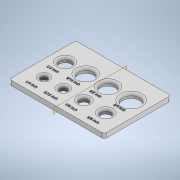
# Autodesk Inventor part: inchHexSocketSetOf8
Saved by Autodesk Inventor 2020.3 (Build 243373000, 373)
## iProperties
Created: 2020-03-13
Part Number: inchHexSocketSetOf8
Material: Generic
Document SubType Name: Modeling
Designer: robst
Density: 1 g/cm^3
Appearance: Default
Author: robst
Autodesk Inventor part; units mm, degrees
(part 1 of 2)
ref_plane "XZ Plane" through (0, 0, 0) normal (0, 1, 0) x (-1, 0, 0)
ref_plane "XY Plane" through (0, 0, 0) normal (0, 0, 1) x (1, 0, 0)
sketch "Sketch1" plane through (0, 0, 0) normal (0, 1, 0) x (-1, 0, 0)
  line L0 (63.5, 44.45) -> (-63.5, 44.45)
  line L1 (-63.5, 44.45) -> (-63.5, -44.45)
  line L2 (-63.5, -44.45) -> (63.5, -44.45)
  line L3 (63.5, -44.45) -> (63.5, 44.45)
  line L4 (63.5, 44.45) -> (-63.5, -44.45) construction
  line L5 (-63.5, 44.45) -> (63.5, -44.45) construction
  point P0 (0, 0)
  dimension "d3" = 88.9
  dimension "d13" = 127
  constraints: 12 end point, 2 midpoint, 2 parallel, 1 horizontal, 1 perpendicular
  measures "d3" distance of L2.end L0.start
  measures "d13" distance of L1.end L2.end
extrude "Extrusion1" add sketch "Sketch1" against normal blind 6.35
sketch "Sketch4" plane through (0, 0, 0) normal (0, 1, 0) x (1, 0, 0)
  line L0 (-63.5, -44.45) -> (-63.5, 44.45) construction
  line L1 (-63.5, -19.05) -> (63.5, -19.05) construction
  line L2 (63.5, 44.45) -> (63.5, -44.45) construction
  line L3 (-63.5, -44.45) -> (63.5, -44.45) projected
  circle A0 centre (-42.4637, -19.05) radius 4.318
  circle A1 centre (-16.6014, -19.05) radius 4.826
  circle A2 centre (10.7848, -19.05) radius 5.842
  circle A3 centre (40.0761, -19.05) radius 6.731
  line L4 (-63.5, 12.7) -> (63.5, 12.7) construction
  circle A4 centre (-45.9232, 12.7) radius 7.874
  circle A5 centre (-18.3134, 12.7) radius 10.033
  circle A6 centre (11.3284, 12.7) radius 9.906
  circle A7 centre (42.3672, 12.7) radius 11.43
  point P0 (0, 0)
  dimension "d16" = 25.4
  dimension "hex1_4inchHole" = 8.636
  dimension "gap0" = 16.7183
  dimension "hex5_16inchHole" = 9.652
  dimension "gap1" = 25.8623
  dimension "hex3_8inchHole" = 11.684
  dimension "gap2" = 27.3863
  dimension "gap3" = 29.2913
  dimension "hex7_16inchHole" = 13.462
  dimension "frontToBackRowGap" = 31.75
  dimension "gap5" = 9.7028
  dimension "hex1_2inchHole" = 15.748
  dimension "hex9_16inchHole" = 20.066
  dimension "gap6" = 27.6098
  dimension "hex5_8inchHole" = 19.812
  dimension "gap7" = 29.6418
  dimension "hex3_4inchHole" = 22.86
  dimension "gap8" = 31.0388
  dimension "d37" = 9.7028
  dimension "d57" = 16.6929
  constraints: 12 point on line, 8 centre point, 4 end point, 1 horizontal, 1 perpendicular
  measures "d16" distance between parallel lines of L1 L3
  measures "hex1_4inchHole" diameter of A0
  measures "gap0" distance edge to line of A0 L0
  measures "hex5_16inchHole" diameter of A1
  measures "gap1" distance of A1.centre A0.centre
  measures "hex3_8inchHole" diameter of A2
  measures "gap2" distance of A2.centre A1.centre
  measures "gap3" distance of A3.centre A2.centre
  measures "hex7_16inchHole" diameter of A3
  measures "frontToBackRowGap" distance between parallel lines of L4 L1
  measures "gap5" distance edge to line of A4 L0
  measures "hex1_2inchHole" diameter of A4
  measures "hex9_16inchHole" diameter of A5
  measures "gap6" distance of A5.centre A4.centre
  measures "hex5_8inchHole" diameter of A6
  measures "gap7" distance of A6.centre A5.centre
  measures "hex3_4inchHole" diameter of A7
  measures "gap8" distance of A7.centre A6.centre
  measures "d37" distance edge to line of A7 L2
  measures "d57" distance edge to line of A3 L2
extrude "Extrusion3" cut sketch "Sketch4" against normal through all
sketch "Sketch7" plane through (0, 0, 0) normal (0, 1, 0) x (1, 0, 0)
  circle A0 centre (-42.4637, -19.05) radius 4.318 construction
  line L0 (63.5, -44.45) -> (-63.5, -44.45) construction
  line L1 (-46.7817, -35.6779) -> (-38.1457, -35.6779) construction
  line L2 (-21.4274, -35.6779) -> (-11.7754, -35.6779) construction
  line L3 (4.9428, -35.6779) -> (16.6268, -35.6779) construction
  line L4 (33.3451, -35.6779) -> (46.8071, -35.6779) construction
  line L5 (-53.7972, -3.81) -> (-38.0492, -3.81) construction
  line L6 (-28.3464, -3.9984) -> (-8.2804, -3.9984) construction
  line L7 (1.4224, -3.8276) -> (21.2344, -3.8276) construction
  line L8 (30.9372, -3.6244) -> (55.5752, -3.6244) construction
  line L9 (-21.4274, -35.6779) -> (-21.4274, -19.05) construction
  circle A1 centre (-16.6014, -19.05) radius 4.826 construction
  line L10 (-11.7754, -35.6779) -> (-11.7754, -19.05) construction
  line L11 (-46.7817, -19.05) -> (-46.7817, -35.6779) construction
  line L12 (-38.1457, -35.6779) -> (-38.1457, -19.05) construction
  line L13 (4.9428, -35.6779) -> (4.9428, -19.05) construction
  circle A2 centre (10.7848, -19.05) radius 5.842 construction
  line L14 (16.6268, -35.6779) -> (16.6268, -19.05) construction
  line L15 (46.8071, -35.6779) -> (46.8071, -19.05) construction
  circle A3 centre (40.0761, -19.05) radius 6.731 construction
  line L16 (33.3451, -35.6779) -> (33.3451, -19.05) construction
  circle A4 centre (-45.9232, 12.7) radius 7.874 construction
  line L17 (-53.7972, 12.7) -> (-53.7972, -3.81) construction
  line L18 (-38.0492, 12.7) -> (-38.0492, -3.81) construction
  circle A5 centre (-18.3134, 12.7) radius 10.033 construction
  line L19 (-28.3464, 12.7) -> (-28.3464, -3.9984) construction
  line L20 (-8.2804, 12.7) -> (-8.2804, -3.9984) construction
  circle A6 centre (11.3284, 12.7) radius 9.906 construction
  line L21 (1.4224, 12.7) -> (1.4224, -3.8276) construction
  line L22 (21.2344, 12.7) -> (21.2344, -3.8276) construction
  circle A7 centre (42.3672, 12.7) radius 11.43 construction
  line L23 (30.9372, 12.7) -> (30.9372, -3.6244) construction
  line L24 (55.5752, 12.702) -> (55.5752, -3.6244) construction
  line L25 (-51.5005, -5.334) -> (-52.9874, -5.334)
  line L26 (-52.9874, -5.334) -> (-52.9874, -5.0228)
  line L27 (-52.9874, -5.0228) -> (-52.4342, -5.0228)
  line L28 (-52.4342, -5.0228) -> (-52.4342, -2.9801)
  line L29 (-52.4342, -2.9801) -> (-52.9874, -2.9801)
  line L30 (-52.9874, -2.9801) -> (-52.9874, -2.701)
  spline S0 degree 2 poles (-52.9874, -2.701) (-52.6738, -2.701) (-52.3774, -2.5231) (-52.3576, -2.2761) knots 0 0 0 1 2 2 2
  line L31 (-52.3576, -2.2761) -> (-52.0414, -2.2761)
  line L32 (-52.0414, -2.2761) -> (-52.0414, -5.0228)
  line L33 (-52.0414, -5.0228) -> (-51.5005, -5.0228)
  line L34 (-51.5005, -5.0228) -> (-51.5005, -5.334)
  line L35 (-49.6727, -2.1501) -> (-50.8657, -5.996)
  line L36 (-50.8657, -5.996) -> (-51.2115, -5.996)
  line L37 (-51.2115, -5.996) -> (-50.0234, -2.1501)
  line L38 (-50.0234, -2.1501) -> (-49.6727, -2.1501)
  line L39 (-47.4571, -5.334) -> (-49.3368, -5.334)
  line L40 (-49.3368, -5.334) -> (-49.3368, -4.9017)
  spline S1 degree 2 poles (-49.3368, -4.9017) (-49.1342, -4.7116) (-48.7736, -4.3583) (-48.6007, -4.1682) knots 0 0 0 1 2 2 2
  spline S2 degree 2 poles (-48.6007, -4.1682) (-48.2524, -3.7853) (-47.998, -3.3259) (-47.998, -3.0813) knots 0 0 0 1 2 2 2
  spline S3 degree 2 poles (-47.998, -3.0813) (-47.998, -2.9529) (-48.0771, -2.7602) (-48.1487, -2.6985) knots 0 0 0 1 2 2 2
  spline S4 degree 2 poles (-48.1487, -2.6985) (-48.2203, -2.6367) (-48.408, -2.575) (-48.5217, -2.575) knots 0 0 0 1 2 2 2
  spline S5 degree 2 poles (-48.5217, -2.575) (-48.6303, -2.575) (-48.8526, -2.6293) (-48.9539, -2.6713) knots 0 0 0 1 2 2 2
  spline S6 degree 2 poles (-48.9539, -2.6713) (-49.0404, -2.7059) (-49.2009, -2.8047) (-49.2503, -2.8393) knots 0 0 0 1 2 2 2
  line L41 (-49.2503, -2.8393) -> (-49.2725, -2.8393)
  line L42 (-49.2725, -2.8393) -> (-49.2725, -2.4046)
  spline S7 degree 2 poles (-49.2725, -2.4046) (-49.1466, -2.3428) (-48.6946, -2.2218) (-48.492, -2.2218) knots 0 0 0 1 2 2 2
  spline S8 degree 2 poles (-48.492, -2.2218) (-48.0647, -2.2218) (-47.5831, -2.6738) (-47.5831, -3.0591) knots 0 0 0 1 2 2 2
  spline S9 degree 2 poles (-47.5831, -3.0591) (-47.5831, -3.2394) (-47.667, -3.5408) (-47.7411, -3.6692) knots 0 0 0 1 2 2 2
  spline S10 degree 2 poles (-47.7411, -3.6692) (-47.8152, -3.8026) (-48.0301, -4.0644) (-48.1487, -4.1904) knots 0 0 0 1 2 2 2
  spline S11 degree 2 poles (-48.1487, -4.1904) (-48.3413, -4.4003) (-48.8131, -4.8499) (-48.9539, -4.9808) knots 0 0 0 1 2 2 2
  line L43 (-48.9539, -4.9808) -> (-47.4571, -4.9808)
  line L44 (-47.4571, -4.9808) -> (-47.4571, -5.334)
  line L45 (-45.2909, -5.334) -> (-45.6762, -5.334)
  line L46 (-45.6762, -5.334) -> (-45.6762, -3.0468)
  line L47 (-45.6762, -3.0468) -> (-45.2909, -3.0468)
  line L48 (-45.2909, -3.0468) -> (-45.2909, -5.334)
  line L49 (-45.2637, -2.6664) -> (-45.7009, -2.6664)
  line L50 (-45.7009, -2.6664) -> (-45.7009, -2.2662)
  line L51 (-45.7009, -2.2662) -> (-45.2637, -2.2662)
  line L52 (-45.2637, -2.2662) -> (-45.2637, -2.6664)
  line L53 (-42.9295, -5.334) -> (-43.3149, -5.334)
  line L54 (-43.3149, -5.334) -> (-43.3149, -4.0298)
  spline S12 degree 2 poles (-43.3149, -4.0298) (-43.3149, -3.8718) (-43.3445, -3.6) (-43.389, -3.5185) knots 0 0 0 1 2 2 2
  spline S13 degree 2 poles (-43.389, -3.5185) (-43.4359, -3.4321) (-43.6039, -3.3481) (-43.7471, -3.3481) knots 0 0 0 1 2 2 2
  spline S14 degree 2 poles (-43.7471, -3.3481) (-43.8904, -3.3481) (-44.1942, -3.5012) (-44.3399, -3.6247) knots 0 0 0 1 2 2 2
  line L55 (-44.3399, -3.6247) -> (-44.3399, -5.334)
  line L56 (-44.3399, -5.334) -> (-44.7252, -5.334)
  line L57 (-44.7252, -5.334) -> (-44.7252, -3.0468)
  line L58 (-44.7252, -3.0468) -> (-44.3399, -3.0468)
  line L59 (-44.3399, -3.0468) -> (-44.3399, -3.3012)
  spline S15 degree 2 poles (-44.3399, -3.3012) (-44.167, -3.1456) (-43.8336, -2.9825) (-43.6458, -2.9825) knots 0 0 0 1 2 2 2
  spline S16 degree 2 poles (-43.6458, -2.9825) (-43.3099, -2.9825) (-42.9295, -3.4271) (-42.9295, -3.8495) knots 0 0 0 1 2 2 2
  line L60 (-42.9295, -3.8495) -> (-42.9295, -5.334)
  spline S17 degree 2 poles (-41.4796, -5.3859) (-41.7168, -5.3859) (-42.1095, -5.2401) (-42.2503, -5.0919) knots 0 0 0 1 2 2 2
  spline S18 degree 2 poles (-42.2503, -5.0919) (-42.3911, -4.9462) (-42.5467, -4.4967) (-42.5467, -4.1953) knots 0 0 0 1 2 2 2
  spline S19 degree 2 poles (-42.5467, -4.1953) (-42.5467, -3.894) (-42.3861, -3.4543) (-42.2503, -3.3061) knots 0 0 0 1 2 2 2
  spline S20 degree 2 poles (-42.2503, -3.3061) (-42.1144, -3.1554) (-41.7118, -2.9949) (-41.4796, -2.9949) knots 0 0 0 1 2 2 2
  spline S21 degree 2 poles (-41.4796, -2.9949) (-41.2919, -2.9949) (-40.9412, -3.1011) (-40.8053, -3.1703) knots 0 0 0 1 2 2 2
  line L61 (-40.8053, -3.1703) -> (-40.8053, -3.6025)
  line L62 (-40.8053, -3.6025) -> (-40.8276, -3.6025)
  spline S22 degree 2 poles (-40.8276, -3.6025) (-40.8695, -3.5679) (-40.998, -3.479) (-41.0894, -3.4321) knots 0 0 0 1 2 2 2
  spline S23 degree 2 poles (-41.0894, -3.4321) (-41.1709, -3.3926) (-41.3883, -3.3308) (-41.4871, -3.3308) knots 0 0 0 1 2 2 2
  spline S24 degree 2 poles (-41.4871, -3.3308) (-41.7859, -3.3308) (-42.149, -3.7828) (-42.149, -4.1953) knots 0 0 0 1 2 2 2
  spline S25 degree 2 poles (-42.149, -4.1953) (-42.149, -4.5979) (-41.7983, -5.0499) (-41.4871, -5.0499) knots 0 0 0 1 2 2 2
  spline S26 degree 2 poles (-41.4871, -5.0499) (-41.2993, -5.0499) (-40.9585, -4.8943) (-40.8276, -4.7733) knots 0 0 0 1 2 2 2
  line L63 (-40.8276, -4.7733) -> (-40.8053, -4.7733)
  line L64 (-40.8053, -4.7733) -> (-40.8053, -5.2056)
  spline S27 degree 2 poles (-40.8053, -5.2056) (-40.8621, -5.2327) (-41.035, -5.3093) (-41.1042, -5.3266) knots 0 0 0 1 2 2 2
  spline S28 degree 2 poles (-41.1042, -5.3266) (-41.203, -5.3562) (-41.3586, -5.3859) (-41.4796, -5.3859) knots 0 0 0 1 2 2 2
  line L65 (-38.6589, -5.334) -> (-39.0442, -5.334)
  line L66 (-39.0442, -5.334) -> (-39.0442, -4.0298)
  spline S29 degree 2 poles (-39.0442, -4.0298) (-39.0442, -3.8718) (-39.0738, -3.6) (-39.1183, -3.5185) knots 0 0 0 1 2 2 2
  spline S30 degree 2 poles (-39.1183, -3.5185) (-39.1652, -3.4321) (-39.3332, -3.3481) (-39.4765, -3.3481) knots 0 0 0 1 2 2 2
  spline S31 degree 2 poles (-39.4765, -3.3481) (-39.6197, -3.3481) (-39.9235, -3.5012) (-40.0693, -3.6247) knots 0 0 0 1 2 2 2
  line L67 (-40.0693, -3.6247) -> (-40.0693, -5.334)
  line L68 (-40.0693, -5.334) -> (-40.4546, -5.334)
  line L69 (-40.4546, -5.334) -> (-40.4546, -2.1501)
  line L70 (-40.4546, -2.1501) -> (-40.0693, -2.1501)
  line L71 (-40.0693, -2.1501) -> (-40.0693, -3.3012)
  spline S32 degree 2 poles (-40.0693, -3.3012) (-39.8964, -3.1456) (-39.5629, -2.9825) (-39.3752, -2.9825) knots 0 0 0 1 2 2 2
  spline S33 degree 2 poles (-39.3752, -2.9825) (-39.0393, -2.9825) (-38.6589, -3.4271) (-38.6589, -3.8495) knots 0 0 0 1 2 2 2
  line L72 (-38.6589, -3.8495) -> (-38.6589, -5.334)
  spline S34 degree 2 poles (-26.8448, -3.4649) (-26.8448, -3.2303) (-26.6917, -2.84) (-26.5583, -2.6992) knots 0 0 0 1 2 2 2
  spline S35 degree 2 poles (-26.5583, -2.6992) (-26.4323, -2.5634) (-26.0643, -2.4127) (-25.8766, -2.4127) knots 0 0 0 1 2 2 2
  spline S36 degree 2 poles (-25.8766, -2.4127) (-25.6666, -2.4127) (-25.3258, -2.5535) (-25.1998, -2.6869) knots 0 0 0 1 2 2 2
  spline S37 degree 2 poles (-25.1998, -2.6869) (-25.0417, -2.8548) (-24.8688, -3.3982) (-24.8688, -3.8157) knots 0 0 0 1 2 2 2
  spline S38 degree 2 poles (-24.8688, -3.8157) (-24.8688, -4.1936) (-25.0393, -4.8704) (-25.2047, -5.0951) knots 0 0 0 1 2 2 2
  spline S39 degree 2 poles (-25.2047, -5.0951) (-25.3801, -5.3323) (-25.8741, -5.5817) (-26.2347, -5.5817) knots 0 0 0 1 2 2 2
  spline S40 degree 2 poles (-26.2347, -5.5817) (-26.3163, -5.5817) (-26.5015, -5.5644) (-26.5805, -5.5397) knots 0 0 0 1 2 2 2
  line L73 (-26.5805, -5.5397) -> (-26.5805, -5.147)
  line L74 (-26.5805, -5.147) -> (-26.5608, -5.147)
  spline S41 degree 2 poles (-26.5608, -5.147) (-26.5089, -5.1766) (-26.2916, -5.2285) (-26.1804, -5.2285) knots 0 0 0 1 2 2 2
  spline S42 degree 2 poles (-26.1804, -5.2285) (-25.7803, -5.2285) (-25.3233, -4.6999) (-25.2912, -4.2109) knots 0 0 0 1 2 2 2
  spline S43 degree 2 poles (-25.2912, -4.2109) (-25.4542, -4.322) (-25.7506, -4.4233) (-25.926, -4.4233) knots 0 0 0 1 2 2 2
  spline S44 degree 2 poles (-25.926, -4.4233) (-26.094, -4.4233) (-26.3731, -4.3492) (-26.5139, -4.243) knots 0 0 0 1 2 2 2
  spline S45 degree 2 poles (-26.5139, -4.243) (-26.6769, -4.117) (-26.8448, -3.7342) (-26.8448, -3.4649) knots 0 0 0 1 2 2 2
  spline S46 degree 2 poles (-25.2813, -3.7243) (-25.2813, -3.4155) (-25.3949, -3.0253) (-25.4962, -2.9191) knots 0 0 0 1 2 2 2
  spline S47 degree 2 poles (-25.4962, -2.9191) (-25.5851, -2.8202) (-25.7704, -2.7461) (-25.8791, -2.7461) knots 0 0 0 1 2 2 2
  spline S48 degree 2 poles (-25.8791, -2.7461) (-26.131, -2.7461) (-26.4299, -3.1068) (-26.4299, -3.4476) knots 0 0 0 1 2 2 2
  spline S49 degree 2 poles (-26.4299, -3.4476) (-26.4299, -3.6403) (-26.3311, -3.8898) (-26.2224, -3.9787) knots 0 0 0 1 2 2 2
  spline S50 degree 2 poles (-26.2224, -3.9787) (-26.1434, -4.0429) (-25.9482, -4.0849) (-25.8346, -4.0849) knots 0 0 0 1 2 2 2
  spline S51 degree 2 poles (-25.8346, -4.0849) (-25.7037, -4.0849) (-25.4023, -3.9935) (-25.2887, -3.9169) knots 0 0 0 1 2 2 2
  spline S52 degree 2 poles (-25.2887, -3.9169) (-25.2863, -3.8873) (-25.2813, -3.786) (-25.2813, -3.7243) knots 0 0 0 1 2 2 2
  line L75 (-23.2065, -2.3386) -> (-24.3995, -6.1844)
  line L76 (-24.3995, -6.1844) -> (-24.7453, -6.1844)
  line L77 (-24.7453, -6.1844) -> (-23.5572, -2.3386)
  line L78 (-23.5572, -2.3386) -> (-23.2065, -2.3386)
  line L79 (-21.144, -5.5224) -> (-22.631, -5.5224)
  line L80 (-22.631, -5.5224) -> (-22.631, -5.2112)
  line L81 (-22.631, -5.2112) -> (-22.0777, -5.2112)
  line L82 (-22.0777, -5.2112) -> (-22.0777, -3.1685)
  line L83 (-22.0777, -3.1685) -> (-22.631, -3.1685)
  line L84 (-22.631, -3.1685) -> (-22.631, -2.8894)
  spline S53 degree 2 poles (-22.631, -2.8894) (-22.3173, -2.8894) (-22.0209, -2.7116) (-22.0011, -2.4646) knots 0 0 0 1 2 2 2
  line L85 (-22.0011, -2.4646) -> (-21.685, -2.4646)
  line L86 (-21.685, -2.4646) -> (-21.685, -5.2112)
  line L87 (-21.685, -5.2112) -> (-21.144, -5.2112)
  line L88 (-21.144, -5.2112) -> (-21.144, -5.5224)
  spline S54 degree 2 poles (-18.6567, -4.5344) (-18.6567, -4.7691) (-18.8123, -5.1668) (-18.9433, -5.3001) knots 0 0 0 1 2 2 2
  spline S55 degree 2 poles (-18.9433, -5.3001) (-19.0791, -5.4409) (-19.42, -5.5867) (-19.625, -5.5867) knots 0 0 0 1 2 2 2
  spline S56 degree 2 poles (-19.625, -5.5867) (-19.83, -5.5867) (-20.1684, -5.4483) (-20.2968, -5.31) knots 0 0 0 1 2 2 2
  spline S57 degree 2 poles (-20.2968, -5.31) (-20.4549, -5.1445) (-20.6327, -4.5888) (-20.6327, -4.1837) knots 0 0 0 1 2 2 2
  spline S58 degree 2 poles (-20.6327, -4.1837) (-20.6327, -3.786) (-20.4697, -3.1463) (-20.2993, -2.9092) knots 0 0 0 1 2 2 2
  spline S59 degree 2 poles (-20.2993, -2.9092) (-20.1338, -2.677) (-19.6102, -2.4176) (-19.2668, -2.4176) knots 0 0 0 1 2 2 2
  spline S60 degree 2 poles (-19.2668, -2.4176) (-19.1656, -2.4176) (-18.9877, -2.4374) (-18.921, -2.4596) knots 0 0 0 1 2 2 2
  line L89 (-18.921, -2.4596) -> (-18.921, -2.8524)
  line L90 (-18.921, -2.8524) -> (-18.9383, -2.8524)
  spline S61 degree 2 poles (-18.9383, -2.8524) (-18.9951, -2.8227) (-19.2026, -2.7708) (-19.3212, -2.7708) knots 0 0 0 1 2 2 2
  spline S62 degree 2 poles (-19.3212, -2.7708) (-19.7015, -2.7708) (-20.1684, -3.2846) (-20.2128, -3.7885) knots 0 0 0 1 2 2 2
  spline S63 degree 2 poles (-20.2128, -3.7885) (-20.0671, -3.6872) (-19.7608, -3.5761) (-19.578, -3.5761) knots 0 0 0 1 2 2 2
  spline S64 degree 2 poles (-19.578, -3.5761) (-19.4002, -3.5761) (-19.1334, -3.6477) (-18.9877, -3.7564) knots 0 0 0 1 2 2 2
  spline S65 degree 2 poles (-18.9877, -3.7564) (-18.8198, -3.8824) (-18.6567, -4.2726) (-18.6567, -4.5344) knots 0 0 0 1 2 2 2
  spline S66 degree 2 poles (-19.0717, -4.5517) (-19.0717, -4.364) (-19.1705, -4.1096) (-19.2792, -4.0207) knots 0 0 0 1 2 2 2
  spline S67 degree 2 poles (-19.2792, -4.0207) (-19.3607, -3.9565) (-19.5632, -3.9145) (-19.6694, -3.9145) knots 0 0 0 1 2 2 2
  spline S68 degree 2 poles (-19.6694, -3.9145) (-19.8127, -3.9145) (-20.0819, -4.0009) (-20.2128, -4.0824) knots 0 0 0 1 2 2 2
  spline S69 degree 2 poles (-20.2128, -4.0824) (-20.2153, -4.1269) (-20.2203, -4.2109) (-20.2203, -4.2751) knots 0 0 0 1 2 2 2
  spline S70 degree 2 poles (-20.2203, -4.2751) (-20.2203, -4.5913) (-20.0968, -4.979) (-20.0029, -5.0803) knots 0 0 0 1 2 2 2
  spline S71 degree 2 poles (-20.0029, -5.0803) (-19.9164, -5.1766) (-19.7287, -5.2532) (-19.6225, -5.2532) knots 0 0 0 1 2 2 2
  spline S72 degree 2 poles (-19.6225, -5.2532) (-19.3755, -5.2532) (-19.0717, -4.9025) (-19.0717, -4.5517) knots 0 0 0 1 2 2 2
  line L91 (-16.5375, -5.5224) -> (-16.9228, -5.5224)
  line L92 (-16.9228, -5.5224) -> (-16.9228, -3.2352)
  line L93 (-16.9228, -3.2352) -> (-16.5375, -3.2352)
  line L94 (-16.5375, -3.2352) -> (-16.5375, -5.5224)
  line L95 (-16.5103, -2.8548) -> (-16.9475, -2.8548)
  line L96 (-16.9475, -2.8548) -> (-16.9475, -2.4547)
  line L97 (-16.9475, -2.4547) -> (-16.5103, -2.4547)
  line L98 (-16.5103, -2.4547) -> (-16.5103, -2.8548)
  line L99 (-14.1761, -5.5224) -> (-14.5614, -5.5224)
  line L100 (-14.5614, -5.5224) -> (-14.5614, -4.2183)
  spline S73 degree 2 poles (-14.5614, -4.2183) (-14.5614, -4.0602) (-14.5911, -3.7885) (-14.6355, -3.707) knots 0 0 0 1 2 2 2
  spline S74 degree 2 poles (-14.6355, -3.707) (-14.6825, -3.6205) (-14.8504, -3.5366) (-14.9937, -3.5366) knots 0 0 0 1 2 2 2
  spline S75 degree 2 poles (-14.9937, -3.5366) (-15.137, -3.5366) (-15.4408, -3.6897) (-15.5865, -3.8132) knots 0 0 0 1 2 2 2
  line L101 (-15.5865, -3.8132) -> (-15.5865, -5.5224)
  line L102 (-15.5865, -5.5224) -> (-15.9718, -5.5224)
  line L103 (-15.9718, -5.5224) -> (-15.9718, -3.2352)
  line L104 (-15.9718, -3.2352) -> (-15.5865, -3.2352)
  line L105 (-15.5865, -3.2352) -> (-15.5865, -3.4896)
  spline S76 degree 2 poles (-15.5865, -3.4896) (-15.4136, -3.334) (-15.0801, -3.171) (-14.8924, -3.171) knots 0 0 0 1 2 2 2
  spline S77 degree 2 poles (-14.8924, -3.171) (-14.5565, -3.171) (-14.1761, -3.6156) (-14.1761, -4.038) knots 0 0 0 1 2 2 2
  line L106 (-14.1761, -4.038) -> (-14.1761, -5.5224)
  spline S78 degree 2 poles (-12.7262, -5.5743) (-12.9633, -5.5743) (-13.3561, -5.4286) (-13.4969, -5.2804) knots 0 0 0 1 2 2 2
  spline S79 degree 2 poles (-13.4969, -5.2804) (-13.6377, -5.1347) (-13.7933, -4.6851) (-13.7933, -4.3838) knots 0 0 0 1 2 2 2
  spline S80 degree 2 poles (-13.7933, -4.3838) (-13.7933, -4.0824) (-13.6327, -3.6428) (-13.4969, -3.4946) knots 0 0 0 1 2 2 2
  spline S81 degree 2 poles (-13.4969, -3.4946) (-13.361, -3.3439) (-12.9584, -3.1833) (-12.7262, -3.1833) knots 0 0 0 1 2 2 2
  spline S82 degree 2 poles (-12.7262, -3.1833) (-12.5385, -3.1833) (-12.1878, -3.2896) (-12.0519, -3.3587) knots 0 0 0 1 2 2 2
  line L107 (-12.0519, -3.3587) -> (-12.0519, -3.791)
  line L108 (-12.0519, -3.791) -> (-12.0741, -3.791)
  spline S83 degree 2 poles (-12.0741, -3.791) (-12.1161, -3.7564) (-12.2446, -3.6675) (-12.336, -3.6205) knots 0 0 0 1 2 2 2
  spline S84 degree 2 poles (-12.336, -3.6205) (-12.4175, -3.581) (-12.6348, -3.5193) (-12.7336, -3.5193) knots 0 0 0 1 2 2 2
  spline S85 degree 2 poles (-12.7336, -3.5193) (-13.0325, -3.5193) (-13.3956, -3.9713) (-13.3956, -4.3838) knots 0 0 0 1 2 2 2
  spline S86 degree 2 poles (-13.3956, -4.3838) (-13.3956, -4.7864) (-13.0449, -5.2384) (-12.7336, -5.2384) knots 0 0 0 1 2 2 2
  spline S87 degree 2 poles (-12.7336, -5.2384) (-12.5459, -5.2384) (-12.205, -5.0828) (-12.0741, -4.9618) knots 0 0 0 1 2 2 2
  line L109 (-12.0741, -4.9618) -> (-12.0519, -4.9618)
  line L110 (-12.0519, -4.9618) -> (-12.0519, -5.394)
  spline S88 degree 2 poles (-12.0519, -5.394) (-12.1087, -5.4212) (-12.2816, -5.4977) (-12.3508, -5.515) knots 0 0 0 1 2 2 2
  spline S89 degree 2 poles (-12.3508, -5.515) (-12.4496, -5.5447) (-12.6052, -5.5743) (-12.7262, -5.5743) knots 0 0 0 1 2 2 2
  line L111 (-9.9055, -5.5224) -> (-10.2908, -5.5224)
  line L112 (-10.2908, -5.5224) -> (-10.2908, -4.2183)
  spline S90 degree 2 poles (-10.2908, -4.2183) (-10.2908, -4.0602) (-10.3204, -3.7885) (-10.3649, -3.707) knots 0 0 0 1 2 2 2
  spline S91 degree 2 poles (-10.3649, -3.707) (-10.4118, -3.6205) (-10.5798, -3.5366) (-10.723, -3.5366) knots 0 0 0 1 2 2 2
  spline S92 degree 2 poles (-10.723, -3.5366) (-10.8663, -3.5366) (-11.1701, -3.6897) (-11.3158, -3.8132) knots 0 0 0 1 2 2 2
  line L113 (-11.3158, -3.8132) -> (-11.3158, -5.5224)
  line L114 (-11.3158, -5.5224) -> (-11.7012, -5.5224)
  line L115 (-11.7012, -5.5224) -> (-11.7012, -2.3386)
  line L116 (-11.7012, -2.3386) -> (-11.3158, -2.3386)
  line L117 (-11.3158, -2.3386) -> (-11.3158, -3.4896)
  spline S93 degree 2 poles (-11.3158, -3.4896) (-11.1429, -3.334) (-10.8095, -3.171) (-10.6218, -3.171) knots 0 0 0 1 2 2 2
  spline S94 degree 2 poles (-10.6218, -3.171) (-10.2858, -3.171) (-9.9055, -3.6156) (-9.9055, -4.038) knots 0 0 0 1 2 2 2
  line L118 (-9.9055, -4.038) -> (-9.9055, -5.5224)
  spline S95 degree 2 poles (5.8721, -4.3833) (5.8721, -4.6032) (5.7313, -4.9786) (5.6029, -5.1169) knots 0 0 0 1 2 2 2
  spline S96 degree 2 poles (5.6029, -5.1169) (5.4745, -5.2552) (5.0916, -5.4158) (4.8545, -5.4158) knots 0 0 0 1 2 2 2
  spline S97 degree 2 poles (4.8545, -5.4158) (4.6371, -5.4158) (4.2123, -5.3195) (4.0567, -5.2429) knots 0 0 0 1 2 2 2
  line L119 (4.0567, -5.2429) -> (4.0567, -4.8106)
  line L120 (4.0567, -4.8106) -> (4.0863, -4.8106)
  spline S98 degree 2 poles (4.0863, -4.8106) (4.1332, -4.8452) (4.3086, -4.9341) (4.4148, -4.9737) knots 0 0 0 1 2 2 2
  spline S99 degree 2 poles (4.4148, -4.9737) (4.5359, -5.0157) (4.7359, -5.0626) (4.8619, -5.0626) knots 0 0 0 1 2 2 2
  spline S100 degree 2 poles (4.8619, -5.0626) (4.9854, -5.0626) (5.2176, -4.9737) (5.3016, -4.8773) knots 0 0 0 1 2 2 2
  spline S101 degree 2 poles (5.3016, -4.8773) (5.3781, -4.7859) (5.4572, -4.5439) (5.4572, -4.3809) knots 0 0 0 1 2 2 2
  spline S102 degree 2 poles (5.4572, -4.3809) (5.4572, -4.2178) (5.3683, -4.0104) (5.2843, -3.9412) knots 0 0 0 1 2 2 2
  spline S103 degree 2 poles (5.2843, -3.9412) (5.1978, -3.8646) (4.9409, -3.8004) (4.7853, -3.8004) knots 0 0 0 1 2 2 2
  spline S104 degree 2 poles (4.7853, -3.8004) (4.6174, -3.8004) (4.2839, -3.8523) (4.1826, -3.8745) knots 0 0 0 1 2 2 2
  line L121 (4.1826, -3.8745) -> (4.1826, -2.3036)
  line L122 (4.1826, -2.3036) -> (5.8548, -2.3036)
  line L123 (5.8548, -2.3036) -> (5.8548, -2.6617)
  line L124 (5.8548, -2.6617) -> (4.5754, -2.6617)
  line L125 (4.5754, -2.6617) -> (4.5754, -3.4744)
  spline S105 degree 2 poles (4.5754, -3.4744) (4.6495, -3.4645) (4.7927, -3.4571) (4.852, -3.4571) knots 0 0 0 1 2 2 2
  spline S106 degree 2 poles (4.852, -3.4571) (5.0867, -3.4571) (5.4102, -3.5336) (5.5584, -3.6473) knots 0 0 0 1 2 2 2
  spline S107 degree 2 poles (5.5584, -3.6473) (5.7091, -3.7609) (5.8721, -4.1067) (5.8721, -4.3833) knots 0 0 0 1 2 2 2
  line L126 (7.5789, -2.1677) -> (6.3859, -6.0135)
  line L127 (6.3859, -6.0135) -> (6.0401, -6.0135)
  line L128 (6.0401, -6.0135) -> (7.2282, -2.1677)
  line L129 (7.2282, -2.1677) -> (7.5789, -2.1677)
  spline S108 degree 2 poles (8.8362, -5.4207) (8.6089, -5.4207) (8.2359, -5.2849) (8.105, -5.1589) knots 0 0 0 1 2 2 2
  spline S109 degree 2 poles (8.105, -5.1589) (7.9766, -5.0354) (7.8432, -4.6995) (7.8432, -4.5093) knots 0 0 0 1 2 2 2
  spline S110 degree 2 poles (7.8432, -4.5093) (7.8432, -4.2623) (8.1075, -3.8473) (8.3594, -3.7238) knots 0 0 0 1 2 2 2
  line L130 (8.3594, -3.7238) -> (8.3594, -3.7115)
  spline S111 degree 2 poles (8.3594, -3.7115) (8.1347, -3.5806) (7.9173, -3.2694) (7.9173, -3.0372) knots 0 0 0 1 2 2 2
  spline S112 degree 2 poles (7.9173, -3.0372) (7.9173, -2.6938) (8.436, -2.2344) (8.8362, -2.2344) knots 0 0 0 1 2 2 2
  spline S113 degree 2 poles (8.8362, -2.2344) (9.2511, -2.2344) (9.7525, -2.6691) (9.7525, -3.01) knots 0 0 0 1 2 2 2
  spline S114 degree 2 poles (9.7525, -3.01) (9.7525, -3.215) (9.5129, -3.6152) (9.2882, -3.7288) knots 0 0 0 1 2 2 2
  line L131 (9.2882, -3.7288) -> (9.2882, -3.7411)
  spline S115 degree 2 poles (9.2882, -3.7411) (9.5549, -3.8646) (9.8291, -4.2203) (9.8291, -4.5019) knots 0 0 0 1 2 2 2
  spline S116 degree 2 poles (9.8291, -4.5019) (9.8291, -4.8922) (9.261, -5.4207) (8.8362, -5.4207) knots 0 0 0 1 2 2 2
  spline S117 degree 2 poles (9.4092, -4.5414) (9.4092, -4.3537) (9.261, -4.1314) (9.051, -4.0178) knots 0 0 0 1 2 2 2
  spline S118 degree 2 poles (9.051, -4.0178) (8.9819, -3.9782) (8.7497, -3.8869) (8.604, -3.8276) knots 0 0 0 1 2 2 2
  spline S119 degree 2 poles (8.604, -3.8276) (8.436, -3.9387) (8.2557, -4.2697) (8.2557, -4.4797) knots 0 0 0 1 2 2 2
  spline S120 degree 2 poles (8.2557, -4.4797) (8.2557, -4.7563) (8.5892, -5.1169) (8.8411, -5.1169) knots 0 0 0 1 2 2 2
  spline S121 degree 2 poles (8.8411, -5.1169) (9.098, -5.1169) (9.4092, -4.8082) (9.4092, -4.5414) knots 0 0 0 1 2 2 2
  spline S122 degree 2 poles (9.3524, -3.0149) (9.3524, -2.8099) (9.0782, -2.5358) (8.8337, -2.5358) knots 0 0 0 1 2 2 2
  spline S123 degree 2 poles (8.8337, -2.5358) (8.6114, -2.5358) (8.3273, -2.7803) (8.3273, -2.9902) knots 0 0 0 1 2 2 2
  spline S124 degree 2 poles (8.3273, -2.9902) (8.3273, -3.1409) (8.4731, -3.3509) (8.6188, -3.4348) knots 0 0 0 1 2 2 2
  spline S125 degree 2 poles (8.6188, -3.4348) (8.6805, -3.4694) (8.9424, -3.5905) (9.0486, -3.625) knots 0 0 0 1 2 2 2
  spline S126 degree 2 poles (9.0486, -3.625) (9.2264, -3.4892) (9.3524, -3.2002) (9.3524, -3.0149) knots 0 0 0 1 2 2 2
  line L132 (11.9607, -5.3516) -> (11.5754, -5.3516)
  line L133 (11.5754, -5.3516) -> (11.5754, -3.0643)
  line L134 (11.5754, -3.0643) -> (11.9607, -3.0643)
  line L135 (11.9607, -3.0643) -> (11.9607, -5.3516)
  line L136 (11.9879, -2.684) -> (11.5507, -2.684)
  line L137 (11.5507, -2.684) -> (11.5507, -2.2838)
  line L138 (11.5507, -2.2838) -> (11.9879, -2.2838)
  line L139 (11.9879, -2.2838) -> (11.9879, -2.684)
  line L140 (14.3221, -5.3516) -> (13.9367, -5.3516)
  line L141 (13.9367, -5.3516) -> (13.9367, -4.0474)
  spline S127 degree 2 poles (13.9367, -4.0474) (13.9367, -3.8893) (13.9071, -3.6176) (13.8626, -3.5361) knots 0 0 0 1 2 2 2
  spline S128 degree 2 poles (13.8626, -3.5361) (13.8157, -3.4497) (13.6477, -3.3657) (13.5045, -3.3657) knots 0 0 0 1 2 2 2
  spline S129 degree 2 poles (13.5045, -3.3657) (13.3612, -3.3657) (13.0574, -3.5188) (12.9117, -3.6423) knots 0 0 0 1 2 2 2
  line L142 (12.9117, -3.6423) -> (12.9117, -5.3516)
  line L143 (12.9117, -5.3516) -> (12.5264, -5.3516)
  line L144 (12.5264, -5.3516) -> (12.5264, -3.0643)
  line L145 (12.5264, -3.0643) -> (12.9117, -3.0643)
  line L146 (12.9117, -3.0643) -> (12.9117, -3.3188)
  spline S130 degree 2 poles (12.9117, -3.3188) (13.0846, -3.1631) (13.418, -3.0001) (13.6058, -3.0001) knots 0 0 0 1 2 2 2
  spline S131 degree 2 poles (13.6058, -3.0001) (13.9417, -3.0001) (14.3221, -3.4447) (14.3221, -3.8671) knots 0 0 0 1 2 2 2
  line L147 (14.3221, -3.8671) -> (14.3221, -5.3516)
  spline S132 degree 2 poles (15.772, -5.4034) (15.5348, -5.4034) (15.1421, -5.2577) (15.0013, -5.1095) knots 0 0 0 1 2 2 2
  spline S133 degree 2 poles (15.0013, -5.1095) (14.8605, -4.9638) (14.7049, -4.5142) (14.7049, -4.2129) knots 0 0 0 1 2 2 2
  spline S134 degree 2 poles (14.7049, -4.2129) (14.7049, -3.9116) (14.8655, -3.4719) (15.0013, -3.3237) knots 0 0 0 1 2 2 2
  spline S135 degree 2 poles (15.0013, -3.3237) (15.1372, -3.173) (15.5398, -3.0125) (15.772, -3.0125) knots 0 0 0 1 2 2 2
  spline S136 degree 2 poles (15.772, -3.0125) (15.9597, -3.0125) (16.3104, -3.1187) (16.4463, -3.1878) knots 0 0 0 1 2 2 2
  line L148 (16.4463, -3.1878) -> (16.4463, -3.6201)
  line L149 (16.4463, -3.6201) -> (16.424, -3.6201)
  spline S137 degree 2 poles (16.424, -3.6201) (16.3821, -3.5855) (16.2536, -3.4966) (16.1622, -3.4497) knots 0 0 0 1 2 2 2
  spline S138 degree 2 poles (16.1622, -3.4497) (16.0807, -3.4101) (15.8633, -3.3484) (15.7645, -3.3484) knots 0 0 0 1 2 2 2
  spline S139 degree 2 poles (15.7645, -3.3484) (15.4657, -3.3484) (15.1026, -3.8004) (15.1026, -4.2129) knots 0 0 0 1 2 2 2
  spline S140 degree 2 poles (15.1026, -4.2129) (15.1026, -4.6155) (15.4533, -5.0675) (15.7645, -5.0675) knots 0 0 0 1 2 2 2
  spline S141 degree 2 poles (15.7645, -5.0675) (15.9523, -5.0675) (16.2931, -4.9119) (16.424, -4.7909) knots 0 0 0 1 2 2 2
  line L150 (16.424, -4.7909) -> (16.4463, -4.7909)
  line L151 (16.4463, -4.7909) -> (16.4463, -5.2231)
  spline S142 degree 2 poles (16.4463, -5.2231) (16.3895, -5.2503) (16.2166, -5.3269) (16.1474, -5.3442) knots 0 0 0 1 2 2 2
  spline S143 degree 2 poles (16.1474, -5.3442) (16.0486, -5.3738) (15.893, -5.4034) (15.772, -5.4034) knots 0 0 0 1 2 2 2
  line L152 (18.5927, -5.3516) -> (18.2074, -5.3516)
  line L153 (18.2074, -5.3516) -> (18.2074, -4.0474)
  spline S144 degree 2 poles (18.2074, -4.0474) (18.2074, -3.8893) (18.1778, -3.6176) (18.1333, -3.5361) knots 0 0 0 1 2 2 2
  spline S145 degree 2 poles (18.1333, -3.5361) (18.0864, -3.4497) (17.9184, -3.3657) (17.7751, -3.3657) knots 0 0 0 1 2 2 2
  spline S146 degree 2 poles (17.7751, -3.3657) (17.6319, -3.3657) (17.3281, -3.5188) (17.1823, -3.6423) knots 0 0 0 1 2 2 2
  line L154 (17.1823, -3.6423) -> (17.1823, -5.3516)
  line L155 (17.1823, -5.3516) -> (16.797, -5.3516)
  line L156 (16.797, -5.3516) -> (16.797, -2.1677)
  line L157 (16.797, -2.1677) -> (17.1823, -2.1677)
  line L158 (17.1823, -2.1677) -> (17.1823, -3.3188)
  spline S147 degree 2 poles (17.1823, -3.3188) (17.3552, -3.1631) (17.6887, -3.0001) (17.8764, -3.0001) knots 0 0 0 1 2 2 2
  spline S148 degree 2 poles (17.8764, -3.0001) (18.2123, -3.0001) (18.5927, -3.4447) (18.5927, -3.8671) knots 0 0 0 1 2 2 2
  line L159 (18.5927, -3.8671) -> (18.5927, -5.3516)
  spline S149 degree 2 poles (36.7749, -2.3894) (36.6637, -2.3894) (36.4439, -2.4437) (36.3377, -2.4857) knots 0 0 0 1 2 2 2
  spline S150 degree 2 poles (36.3377, -2.4857) (36.2389, -2.5277) (36.0932, -2.6166) (36.0363, -2.6562) knots 0 0 0 1 2 2 2
  line L160 (36.0363, -2.6562) -> (36.0116, -2.6562)
  line L161 (36.0116, -2.6562) -> (36.0116, -2.2239)
  spline S151 degree 2 poles (36.0116, -2.2239) (36.145, -2.1523) (36.602, -2.0362) (36.807, -2.0362) knots 0 0 0 1 2 2 2
  spline S152 degree 2 poles (36.807, -2.0362) (37.0145, -2.0362) (37.3232, -2.1202) (37.4492, -2.2091) knots 0 0 0 1 2 2 2
  spline S153 degree 2 poles (37.4492, -2.2091) (37.5826, -2.3054) (37.7209, -2.5845) (37.7209, -2.7723) knots 0 0 0 1 2 2 2
  spline S154 degree 2 poles (37.7209, -2.7723) (37.7209, -3.0242) (37.3899, -3.4046) (37.1577, -3.454) knots 0 0 0 1 2 2 2
  line L162 (37.1577, -3.454) -> (37.1577, -3.4836)
  spline S155 degree 2 poles (37.1577, -3.4836) (37.2541, -3.5034) (37.4739, -3.5923) (37.5678, -3.6812) knots 0 0 0 1 2 2 2
  spline S156 degree 2 poles (37.5678, -3.6812) (37.6616, -3.7677) (37.7802, -4.0443) (37.7802, -4.2444) knots 0 0 0 1 2 2 2
  spline S157 degree 2 poles (37.7802, -4.2444) (37.7802, -4.4494) (37.6394, -4.7977) (37.5109, -4.931) knots 0 0 0 1 2 2 2
  spline S158 degree 2 poles (37.5109, -4.931) (37.3776, -5.0694) (36.9996, -5.2126) (36.7601, -5.2126) knots 0 0 0 1 2 2 2
  spline S159 degree 2 poles (36.7601, -5.2126) (36.5303, -5.2126) (36.0808, -5.1015) (35.9277, -5.0249) knots 0 0 0 1 2 2 2
  line L163 (35.9277, -5.0249) -> (35.9277, -4.5927)
  line L164 (35.9277, -4.5927) -> (35.9573, -4.5927)
  spline S160 degree 2 poles (35.9573, -4.5927) (36.0857, -4.6865) (36.5205, -4.8594) (36.7354, -4.8594) knots 0 0 0 1 2 2 2
  spline S161 degree 2 poles (36.7354, -4.8594) (36.8613, -4.8594) (37.1133, -4.7804) (37.1973, -4.689) knots 0 0 0 1 2 2 2
  spline S162 degree 2 poles (37.1973, -4.689) (37.2788, -4.5976) (37.3652, -4.3802) (37.3652, -4.2147) knots 0 0 0 1 2 2 2
  spline S163 degree 2 poles (37.3652, -4.2147) (37.3652, -4.0492) (37.2689, -3.8344) (37.1824, -3.7726) knots 0 0 0 1 2 2 2
  spline S164 degree 2 poles (37.1824, -3.7726) (37.096, -3.7109) (36.8613, -3.6639) (36.723, -3.6639) knots 0 0 0 1 2 2 2
  line L165 (36.723, -3.6639) -> (36.5501, -3.6639)
  line L166 (36.5501, -3.6639) -> (36.5501, -3.3255)
  line L167 (36.5501, -3.3255) -> (36.686, -3.3255)
  spline S165 degree 2 poles (36.686, -3.3255) (36.9601, -3.3255) (37.3059, -3.0637) (37.3059, -2.8142) knots 0 0 0 1 2 2 2
  spline S166 degree 2 poles (37.3059, -2.8142) (37.3059, -2.6982) (37.217, -2.5327) (37.1454, -2.4833) knots 0 0 0 1 2 2 2
  spline S167 degree 2 poles (37.1454, -2.4833) (37.0688, -2.4314) (36.8811, -2.3894) (36.7749, -2.3894) knots 0 0 0 1 2 2 2
  line L168 (39.5067, -1.9646) -> (38.3137, -5.8104)
  line L169 (38.3137, -5.8104) -> (37.9679, -5.8104)
  line L170 (37.9679, -5.8104) -> (39.156, -1.9646)
  line L171 (39.156, -1.9646) -> (39.5067, -1.9646)
  line L172 (41.8038, -4.1011) -> (41.4407, -4.1011)
  line L173 (41.4407, -4.1011) -> (41.4407, -5.1484)
  line L174 (41.4407, -5.1484) -> (41.048, -5.1484)
  line L175 (41.048, -5.1484) -> (41.048, -4.1011)
  line L176 (41.048, -4.1011) -> (39.7018, -4.1011)
  line L177 (39.7018, -4.1011) -> (39.7018, -3.6713)
  line L178 (39.7018, -3.6713) -> (41.0653, -2.1004)
  line L179 (41.0653, -2.1004) -> (41.4407, -2.1004)
  line L180 (41.4407, -2.1004) -> (41.4407, -3.7726)
  line L181 (41.4407, -3.7726) -> (41.8038, -3.7726)
  line L182 (41.8038, -3.7726) -> (41.8038, -4.1011)
  line L183 (41.048, -3.7726) -> (41.048, -2.5821)
  line L184 (41.048, -2.5821) -> (40.0229, -3.7726)
  line L185 (40.0229, -3.7726) -> (41.048, -3.7726)
  line L186 (43.8885, -5.1484) -> (43.5032, -5.1484)
  line L187 (43.5032, -5.1484) -> (43.5032, -2.8612)
  line L188 (43.5032, -2.8612) -> (43.8885, -2.8612)
  line L189 (43.8885, -2.8612) -> (43.8885, -5.1484)
  line L190 (43.9157, -2.4808) -> (43.4785, -2.4808)
  line L191 (43.4785, -2.4808) -> (43.4785, -2.0806)
  line L192 (43.4785, -2.0806) -> (43.9157, -2.0806)
  line L193 (43.9157, -2.0806) -> (43.9157, -2.4808)
  line L194 (46.2499, -5.1484) -> (45.8645, -5.1484)
  line L195 (45.8645, -5.1484) -> (45.8645, -3.8442)
  spline S168 degree 2 poles (45.8645, -3.8442) (45.8645, -3.6862) (45.8349, -3.4145) (45.7904, -3.3329) knots 0 0 0 1 2 2 2
  spline S169 degree 2 poles (45.7904, -3.3329) (45.7435, -3.2465) (45.5755, -3.1625) (45.4323, -3.1625) knots 0 0 0 1 2 2 2
  spline S170 degree 2 poles (45.4323, -3.1625) (45.289, -3.1625) (44.9852, -3.3157) (44.8395, -3.4392) knots 0 0 0 1 2 2 2
  line L196 (44.8395, -3.4392) -> (44.8395, -5.1484)
  line L197 (44.8395, -5.1484) -> (44.4542, -5.1484)
  line L198 (44.4542, -5.1484) -> (44.4542, -2.8612)
  line L199 (44.4542, -2.8612) -> (44.8395, -2.8612)
  line L200 (44.8395, -2.8612) -> (44.8395, -3.1156)
  spline S171 degree 2 poles (44.8395, -3.1156) (45.0124, -2.96) (45.3458, -2.797) (45.5336, -2.797) knots 0 0 0 1 2 2 2
  spline S172 degree 2 poles (45.5336, -2.797) (45.8695, -2.797) (46.2499, -3.2416) (46.2499, -3.6639) knots 0 0 0 1 2 2 2
  line L201 (46.2499, -3.6639) -> (46.2499, -5.1484)
  spline S173 degree 2 poles (47.6998, -5.2003) (47.4626, -5.2003) (47.0699, -5.0545) (46.9291, -4.9063) knots 0 0 0 1 2 2 2
  spline S174 degree 2 poles (46.9291, -4.9063) (46.7883, -4.7606) (46.6327, -4.3111) (46.6327, -4.0097) knots 0 0 0 1 2 2 2
  spline S175 degree 2 poles (46.6327, -4.0097) (46.6327, -3.7084) (46.7933, -3.2687) (46.9291, -3.1205) knots 0 0 0 1 2 2 2
  spline S176 degree 2 poles (46.9291, -3.1205) (47.065, -2.9699) (47.4676, -2.8093) (47.6998, -2.8093) knots 0 0 0 1 2 2 2
  spline S177 degree 2 poles (47.6998, -2.8093) (47.8875, -2.8093) (48.2382, -2.9155) (48.3741, -2.9847) knots 0 0 0 1 2 2 2
  line L202 (48.3741, -2.9847) -> (48.3741, -3.4169)
  line L203 (48.3741, -3.4169) -> (48.3518, -3.4169)
  spline S178 degree 2 poles (48.3518, -3.4169) (48.3099, -3.3823) (48.1814, -3.2934) (48.09, -3.2465) knots 0 0 0 1 2 2 2
  spline S179 degree 2 poles (48.09, -3.2465) (48.0085, -3.207) (47.7911, -3.1452) (47.6923, -3.1452) knots 0 0 0 1 2 2 2
  spline S180 degree 2 poles (47.6923, -3.1452) (47.3935, -3.1452) (47.0304, -3.5972) (47.0304, -4.0097) knots 0 0 0 1 2 2 2
  spline S181 degree 2 poles (47.0304, -4.0097) (47.0304, -4.4123) (47.3811, -4.8644) (47.6923, -4.8644) knots 0 0 0 1 2 2 2
  spline S182 degree 2 poles (47.6923, -4.8644) (47.8801, -4.8644) (48.2209, -4.7087) (48.3518, -4.5877) knots 0 0 0 1 2 2 2
  line L204 (48.3518, -4.5877) -> (48.3741, -4.5877)
  line L205 (48.3741, -4.5877) -> (48.3741, -5.02)
  spline S183 degree 2 poles (48.3741, -5.02) (48.3173, -5.0471) (48.1444, -5.1237) (48.0752, -5.141) knots 0 0 0 1 2 2 2
  spline S184 degree 2 poles (48.0752, -5.141) (47.9764, -5.1706) (47.8208, -5.2003) (47.6998, -5.2003) knots 0 0 0 1 2 2 2
  line L206 (50.5205, -5.1484) -> (50.1352, -5.1484)
  line L207 (50.1352, -5.1484) -> (50.1352, -3.8442)
  spline S185 degree 2 poles (50.1352, -3.8442) (50.1352, -3.6862) (50.1056, -3.4145) (50.0611, -3.3329) knots 0 0 0 1 2 2 2
  spline S186 degree 2 poles (50.0611, -3.3329) (50.0142, -3.2465) (49.8462, -3.1625) (49.7029, -3.1625) knots 0 0 0 1 2 2 2
  spline S187 degree 2 poles (49.7029, -3.1625) (49.5597, -3.1625) (49.2559, -3.3157) (49.1101, -3.4392) knots 0 0 0 1 2 2 2
  line L208 (49.1101, -3.4392) -> (49.1101, -5.1484)
  line L209 (49.1101, -5.1484) -> (48.7248, -5.1484)
  line L210 (48.7248, -5.1484) -> (48.7248, -1.9646)
  line L211 (48.7248, -1.9646) -> (49.1101, -1.9646)
  line L212 (49.1101, -1.9646) -> (49.1101, -3.1156)
  spline S188 degree 2 poles (49.1101, -3.1156) (49.283, -2.96) (49.6165, -2.797) (49.8042, -2.797) knots 0 0 0 1 2 2 2
  spline S189 degree 2 poles (49.8042, -2.797) (50.1401, -2.797) (50.5205, -3.2416) (50.5205, -3.6639) knots 0 0 0 1 2 2 2
  line L213 (50.5205, -3.6639) -> (50.5205, -5.1484)
  line L214 (-48.041, -37.2019) -> (-49.528, -37.2019)
  line L215 (-49.528, -37.2019) -> (-49.528, -36.8906)
  line L216 (-49.528, -36.8906) -> (-48.9747, -36.8906)
  line L217 (-48.9747, -36.8906) -> (-48.9747, -34.8479)
  line L218 (-48.9747, -34.8479) -> (-49.528, -34.8479)
  line L219 (-49.528, -34.8479) -> (-49.528, -34.5688)
  spline S190 degree 2 poles (-49.528, -34.5688) (-49.2143, -34.5688) (-48.9179, -34.391) (-48.8981, -34.144) knots 0 0 0 1 2 2 2
  line L220 (-48.8981, -34.144) -> (-48.582, -34.144)
  line L221 (-48.582, -34.144) -> (-48.582, -36.8906)
  line L222 (-48.582, -36.8906) -> (-48.041, -36.8906)
  line L223 (-48.041, -36.8906) -> (-48.041, -37.2019)
  line L224 (-46.2132, -34.018) -> (-47.4062, -37.8638)
  line L225 (-47.4062, -37.8638) -> (-47.752, -37.8638)
  line L226 (-47.752, -37.8638) -> (-46.5639, -34.018)
  line L227 (-46.5639, -34.018) -> (-46.2132, -34.018)
  line L228 (-43.9161, -36.1546) -> (-44.2792, -36.1546)
  line L229 (-44.2792, -36.1546) -> (-44.2792, -37.2019)
  line L230 (-44.2792, -37.2019) -> (-44.6719, -37.2019)
  line L231 (-44.6719, -37.2019) -> (-44.6719, -36.1546)
  line L232 (-44.6719, -36.1546) -> (-46.0181, -36.1546)
  line L233 (-46.0181, -36.1546) -> (-46.0181, -35.7248)
  line L234 (-46.0181, -35.7248) -> (-44.6546, -34.1539)
  line L235 (-44.6546, -34.1539) -> (-44.2792, -34.1539)
  line L236 (-44.2792, -34.1539) -> (-44.2792, -35.8261)
  line L237 (-44.2792, -35.8261) -> (-43.9161, -35.8261)
  line L238 (-43.9161, -35.8261) -> (-43.9161, -36.1546)
  line L239 (-44.6719, -35.8261) -> (-44.6719, -34.6355)
  line L240 (-44.6719, -34.6355) -> (-45.697, -35.8261)
  line L241 (-45.697, -35.8261) -> (-44.6719, -35.8261)
  line L242 (-41.8314, -37.2019) -> (-42.2167, -37.2019)
  line L243 (-42.2167, -37.2019) -> (-42.2167, -34.9146)
  line L244 (-42.2167, -34.9146) -> (-41.8314, -34.9146)
  line L245 (-41.8314, -34.9146) -> (-41.8314, -37.2019)
  line L246 (-41.8042, -34.5342) -> (-42.2414, -34.5342)
  line L247 (-42.2414, -34.5342) -> (-42.2414, -34.1341)
  line L248 (-42.2414, -34.1341) -> (-41.8042, -34.1341)
  line L249 (-41.8042, -34.1341) -> (-41.8042, -34.5342)
  line L250 (-39.4701, -37.2019) -> (-39.8554, -37.2019)
  line L251 (-39.8554, -37.2019) -> (-39.8554, -35.8977)
  spline S191 degree 2 poles (-39.8554, -35.8977) (-39.8554, -35.7396) (-39.885, -35.4679) (-39.9295, -35.3864) knots 0 0 0 1 2 2 2
  spline S192 degree 2 poles (-39.9295, -35.3864) (-39.9764, -35.3) (-40.1444, -35.216) (-40.2876, -35.216) knots 0 0 0 1 2 2 2
  spline S193 degree 2 poles (-40.2876, -35.216) (-40.4309, -35.216) (-40.7347, -35.3691) (-40.8804, -35.4926) knots 0 0 0 1 2 2 2
  line L252 (-40.8804, -35.4926) -> (-40.8804, -37.2019)
  line L253 (-40.8804, -37.2019) -> (-41.2658, -37.2019)
  line L254 (-41.2658, -37.2019) -> (-41.2658, -34.9146)
  line L255 (-41.2658, -34.9146) -> (-40.8804, -34.9146)
  line L256 (-40.8804, -34.9146) -> (-40.8804, -35.169)
  spline S194 degree 2 poles (-40.8804, -35.169) (-40.7075, -35.0134) (-40.3741, -34.8504) (-40.1864, -34.8504) knots 0 0 0 1 2 2 2
  spline S195 degree 2 poles (-40.1864, -34.8504) (-39.8504, -34.8504) (-39.4701, -35.295) (-39.4701, -35.7174) knots 0 0 0 1 2 2 2
  line L257 (-39.4701, -35.7174) -> (-39.4701, -37.2019)
  spline S196 degree 2 poles (-38.0202, -37.2537) (-38.2573, -37.2537) (-38.65, -37.108) (-38.7908, -36.9598) knots 0 0 0 1 2 2 2
  spline S197 degree 2 poles (-38.7908, -36.9598) (-38.9316, -36.8141) (-39.0872, -36.3645) (-39.0872, -36.0632) knots 0 0 0 1 2 2 2
  spline S198 degree 2 poles (-39.0872, -36.0632) (-39.0872, -35.7618) (-38.9267, -35.3222) (-38.7908, -35.174) knots 0 0 0 1 2 2 2
  spline S199 degree 2 poles (-38.7908, -35.174) (-38.655, -35.0233) (-38.2523, -34.8628) (-38.0202, -34.8628) knots 0 0 0 1 2 2 2
  spline S200 degree 2 poles (-38.0202, -34.8628) (-37.8324, -34.8628) (-37.4817, -34.969) (-37.3458, -35.0381) knots 0 0 0 1 2 2 2
  line L258 (-37.3458, -35.0381) -> (-37.3458, -35.4704)
  line L259 (-37.3458, -35.4704) -> (-37.3681, -35.4704)
  spline S201 degree 2 poles (-37.3681, -35.4704) (-37.4101, -35.4358) (-37.5385, -35.3469) (-37.6299, -35.3) knots 0 0 0 1 2 2 2
  spline S202 degree 2 poles (-37.6299, -35.3) (-37.7114, -35.2604) (-37.9288, -35.1987) (-38.0276, -35.1987) knots 0 0 0 1 2 2 2
  spline S203 degree 2 poles (-38.0276, -35.1987) (-38.3264, -35.1987) (-38.6895, -35.6507) (-38.6895, -36.0632) knots 0 0 0 1 2 2 2
  spline S204 degree 2 poles (-38.6895, -36.0632) (-38.6895, -36.4658) (-38.3388, -36.9178) (-38.0276, -36.9178) knots 0 0 0 1 2 2 2
  spline S205 degree 2 poles (-38.0276, -36.9178) (-37.8399, -36.9178) (-37.499, -36.7622) (-37.3681, -36.6412) knots 0 0 0 1 2 2 2
  line L260 (-37.3681, -36.6412) -> (-37.3458, -36.6412)
  line L261 (-37.3458, -36.6412) -> (-37.3458, -37.0734)
  spline S206 degree 2 poles (-37.3458, -37.0734) (-37.4027, -37.1006) (-37.5756, -37.1772) (-37.6447, -37.1945) knots 0 0 0 1 2 2 2
  spline S207 degree 2 poles (-37.6447, -37.1945) (-37.7435, -37.2241) (-37.8991, -37.2537) (-38.0202, -37.2537) knots 0 0 0 1 2 2 2
  line L262 (-35.1994, -37.2019) -> (-35.5847, -37.2019)
  line L263 (-35.5847, -37.2019) -> (-35.5847, -35.8977)
  spline S208 degree 2 poles (-35.5847, -35.8977) (-35.5847, -35.7396) (-35.6144, -35.4679) (-35.6588, -35.3864) knots 0 0 0 1 2 2 2
  spline S209 degree 2 poles (-35.6588, -35.3864) (-35.7058, -35.3) (-35.8737, -35.216) (-36.017, -35.216) knots 0 0 0 1 2 2 2
  spline S210 degree 2 poles (-36.017, -35.216) (-36.1602, -35.216) (-36.4641, -35.3691) (-36.6098, -35.4926) knots 0 0 0 1 2 2 2
  line L264 (-36.6098, -35.4926) -> (-36.6098, -37.2019)
  line L265 (-36.6098, -37.2019) -> (-36.9951, -37.2019)
  line L266 (-36.9951, -37.2019) -> (-36.9951, -34.018)
  line L267 (-36.9951, -34.018) -> (-36.6098, -34.018)
  line L268 (-36.6098, -34.018) -> (-36.6098, -35.169)
  spline S211 degree 2 poles (-36.6098, -35.169) (-36.4369, -35.0134) (-36.1034, -34.8504) (-35.9157, -34.8504) knots 0 0 0 1 2 2 2
  spline S212 degree 2 poles (-35.9157, -34.8504) (-35.5798, -34.8504) (-35.1994, -35.295) (-35.1994, -35.7174) knots 0 0 0 1 2 2 2
  line L269 (-35.1994, -35.7174) -> (-35.1994, -37.2019)
  spline S213 degree 2 poles (-23.2013, -36.2336) (-23.2013, -36.4535) (-23.3421, -36.8289) (-23.4706, -36.9672) knots 0 0 0 1 2 2 2
  spline S214 degree 2 poles (-23.4706, -36.9672) (-23.599, -37.1055) (-23.9818, -37.2661) (-24.219, -37.2661) knots 0 0 0 1 2 2 2
  spline S215 degree 2 poles (-24.219, -37.2661) (-24.4363, -37.2661) (-24.8612, -37.1698) (-25.0168, -37.0932) knots 0 0 0 1 2 2 2
  line L270 (-25.0168, -37.0932) -> (-25.0168, -36.6609)
  line L271 (-25.0168, -36.6609) -> (-24.9871, -36.6609)
  spline S216 degree 2 poles (-24.9871, -36.6609) (-24.9402, -36.6955) (-24.7648, -36.7844) (-24.6586, -36.824) knots 0 0 0 1 2 2 2
  spline S217 degree 2 poles (-24.6586, -36.824) (-24.5376, -36.8659) (-24.3375, -36.9129) (-24.2116, -36.9129) knots 0 0 0 1 2 2 2
  spline S218 degree 2 poles (-24.2116, -36.9129) (-24.0881, -36.9129) (-23.8559, -36.824) (-23.7719, -36.7276) knots 0 0 0 1 2 2 2
  spline S219 degree 2 poles (-23.7719, -36.7276) (-23.6953, -36.6362) (-23.6163, -36.3942) (-23.6163, -36.2312) knots 0 0 0 1 2 2 2
  spline S220 degree 2 poles (-23.6163, -36.2312) (-23.6163, -36.0681) (-23.7052, -35.8606) (-23.7892, -35.7915) knots 0 0 0 1 2 2 2
  spline S221 degree 2 poles (-23.7892, -35.7915) (-23.8756, -35.7149) (-24.1325, -35.6507) (-24.2881, -35.6507) knots 0 0 0 1 2 2 2
  spline S222 degree 2 poles (-24.2881, -35.6507) (-24.4561, -35.6507) (-24.7895, -35.7026) (-24.8908, -35.7248) knots 0 0 0 1 2 2 2
  line L272 (-24.8908, -35.7248) -> (-24.8908, -34.1539)
  line L273 (-24.8908, -34.1539) -> (-23.2186, -34.1539)
  line L274 (-23.2186, -34.1539) -> (-23.2186, -34.512)
  line L275 (-23.2186, -34.512) -> (-24.4981, -34.512)
  line L276 (-24.4981, -34.512) -> (-24.4981, -35.3247)
  spline S223 degree 2 poles (-24.4981, -35.3247) (-24.424, -35.3148) (-24.2807, -35.3074) (-24.2214, -35.3074) knots 0 0 0 1 2 2 2
  spline S224 degree 2 poles (-24.2214, -35.3074) (-23.9868, -35.3074) (-23.6632, -35.3839) (-23.515, -35.4976) knots 0 0 0 1 2 2 2
  spline S225 degree 2 poles (-23.515, -35.4976) (-23.3643, -35.6112) (-23.2013, -35.957) (-23.2013, -36.2336) knots 0 0 0 1 2 2 2
  line L277 (-21.4945, -34.018) -> (-22.6876, -37.8638)
  line L278 (-22.6876, -37.8638) -> (-23.0334, -37.8638)
  line L279 (-23.0334, -37.8638) -> (-21.8453, -34.018)
  line L280 (-21.8453, -34.018) -> (-21.4945, -34.018)
  line L281 (-19.4321, -37.2019) -> (-20.919, -37.2019)
  line L282 (-20.919, -37.2019) -> (-20.919, -36.8906)
  line L283 (-20.919, -36.8906) -> (-20.3657, -36.8906)
  line L284 (-20.3657, -36.8906) -> (-20.3657, -34.8479)
  line L285 (-20.3657, -34.8479) -> (-20.919, -34.8479)
  line L286 (-20.919, -34.8479) -> (-20.919, -34.5688)
  spline S226 degree 2 poles (-20.919, -34.5688) (-20.6053, -34.5688) (-20.3089, -34.391) (-20.2892, -34.144) knots 0 0 0 1 2 2 2
  line L287 (-20.2892, -34.144) -> (-19.973, -34.144)
  line L288 (-19.973, -34.144) -> (-19.973, -36.8906)
  line L289 (-19.973, -36.8906) -> (-19.4321, -36.8906)
  line L290 (-19.4321, -36.8906) -> (-19.4321, -37.2019)
  spline S227 degree 2 poles (-16.9448, -36.2139) (-16.9448, -36.4485) (-17.1004, -36.8462) (-17.2313, -36.9796) knots 0 0 0 1 2 2 2
  spline S228 degree 2 poles (-17.2313, -36.9796) (-17.3671, -37.1204) (-17.708, -37.2661) (-17.913, -37.2661) knots 0 0 0 1 2 2 2
  spline S229 degree 2 poles (-17.913, -37.2661) (-18.118, -37.2661) (-18.4564, -37.1278) (-18.5849, -36.9894) knots 0 0 0 1 2 2 2
  spline S230 degree 2 poles (-18.5849, -36.9894) (-18.7429, -36.824) (-18.9208, -36.2682) (-18.9208, -35.8631) knots 0 0 0 1 2 2 2
  spline S231 degree 2 poles (-18.9208, -35.8631) (-18.9208, -35.4654) (-18.7578, -34.8257) (-18.5873, -34.5886) knots 0 0 0 1 2 2 2
  spline S232 degree 2 poles (-18.5873, -34.5886) (-18.4218, -34.3564) (-17.8982, -34.0971) (-17.5549, -34.0971) knots 0 0 0 1 2 2 2
  spline S233 degree 2 poles (-17.5549, -34.0971) (-17.4536, -34.0971) (-17.2758, -34.1168) (-17.2091, -34.139) knots 0 0 0 1 2 2 2
  line L291 (-17.2091, -34.139) -> (-17.2091, -34.5318)
  line L292 (-17.2091, -34.5318) -> (-17.2264, -34.5318)